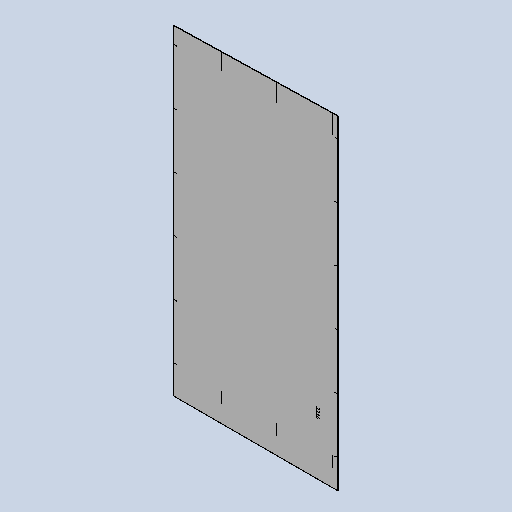
# Autodesk Inventor part: GBK 2231 shield 6
Saved by Autodesk Inventor 2026.2 (Build 302298010, 298A)
## iProperties
Created: 2026-04-17
Part Number: GBK 2231 shield 6
Material: Steel
Document SubType Name: Sheet Metal
Designer: pokla
Stock Number: 2236
Mass: 135011 g
Surface Area: 86345 cm^2
Volume: 17198.8 cm^3
Density: 7.85 g/cm^3
Flat Pattern Width: 148 cm
Flat Pattern Length: 292.2 cm
Flat Pattern Area: 43245.6 cm^2
Sheet Metal Rule: Default_mm
Sheet Metal Width: 1480,000 мм
Sheet Metal Length: 2922,000 мм
Sheet Metal Area: 4324560,000 мм^2
Appearance: Default
Author: admin
Autodesk Inventor part; units mm, degrees
ref_plane "YZ Plane" through (0, 0, 0) normal (1, 0, 0) x (0, 1, 0)
ref_plane "XZ Plane" through (0, 0, 0) normal (0, 1, 0) x (-1, 0, 0)
ref_plane "XY Plane" through (0, 0, 0) normal (0, 0, 1) x (1, 0, 0)
sketch "Sketch1" plane through (0, 0, 0) normal (0, 0, 1) x (1, 0, 0)
  line L0 (740, -1490) -> (-740, -1490)
  line L1 (-740, -1490) -> (-740, 1490)
  line L2 (-740, 1490) -> (740, 1490)
  line L3 (740, 1490) -> (740, -1490)
  line L4 (740, -1490) -> (-740, 1490) construction
  line L5 (-740, -1490) -> (740, 1490) construction
  line L6 (740, 1432) -> (-740, 1398.4141)
  point P0 (0, 0)
  dimension "d0" = 1480
  dimension "d1" = 2980
  dimension "d3" = 1.3
  dimension "d5" = 2922
  measures "d0" distance of L1.end L2.end
  measures "d1" distance of L0.end L1.end
  measures "d3" angle of L2 L6
  measures "d5" distance of L0.start L6.start
extrude "Plate1" add sketch "Sketch1" along normal blind 4 contours L0 L1 L6 L3
sketch "Sketch3" plane through (0, 0, 4) normal (0, 0, 1) x (1, 0, 0)
  line L0 (575.4966, -928.4274) -> (575.4966, -1128.991) construction
  line L1 (575.4966, -1128.991) -> (488.2456, -1128.991) construction
  line L2 (488.2456, -1128.991) -> (488.2456, -928.4274) construction
  line L3 (488.2456, -928.4274) -> (575.4966, -928.4274) construction
  line L4 (690.2486, -1238) -> (690.2486, -1335) projected
  line L5 (690.2486, -1335) -> (686.2496, -1335) projected
  line L6 (190.12, -1238) -> (190.12, -1335) projected
  line L7 (190.12, -1335) -> (186.121, -1335) projected
  line L8 (-310.0086, -1238) -> (-310.0086, -1335) projected
  line L9 (-310.0086, -1335) -> (-314.0076, -1335) projected
  line L10 (-310.0086, 1460.5) -> (-310.0086, 1256.8333) projected
  line L11 (190.12, 1460.5) -> (190.12, 1256.5) projected
  line L12 (690.2486, 1460.5) -> (690.2486, 1256.5) projected
  line L13 (770, 1252.8333) -> (710, 1252.8333) projected
  line L14 (710, 1248.8333) -> (710, 1252.8333) projected
  line L15 (770, 756.1667) -> (710, 756.1667) projected
  line L16 (710, 752.1667) -> (710, 756.1667) projected
  line L17 (770, 259.5) -> (710, 259.5) projected
  line L18 (710, 255.5) -> (710, 259.5) projected
  line L19 (770, -237.1667) -> (710, -237.1667) projected
  line L20 (710, -241.1667) -> (710, -237.1667) projected
  line L21 (770, -733.8333) -> (710, -733.8333) projected
  line L22 (710, -737.8333) -> (710, -733.8333) projected
  line L23 (770, -1230.5) -> (710, -1230.5) projected
  line L24 (710, -1234.5) -> (710, -1230.5) projected
  line L25 (-710, 1252.8333) -> (-739.3197, 1252.8333) projected
  line L26 (-710, 1248.8333) -> (-710, 1252.8333) projected
  line L27 (-710, 756.1667) -> (-739.3197, 756.1667) projected
  line L28 (-710, 752.1667) -> (-710, 756.1667) projected
  line L29 (-710, 259.5) -> (-739.3197, 259.5) projected
  line L30 (-710, 255.5) -> (-710, 259.5) projected
  line L31 (-710, -237.1667) -> (-739.3197, -237.1667) projected
  line L32 (-710, -241.1667) -> (-710, -237.1667) projected
  line L33 (-710, -733.8333) -> (-739.3197, -733.8333) projected
  line L34 (-710, -737.8333) -> (-710, -733.8333) projected
  line L35 (-710, -1230.5) -> (-739.3197, -1230.5) projected
  line L36 (-710, -1234.5) -> (-710, -1230.5) projected
  point P0 (0, 0)
  constraints: 2 other
mark "Mark2"
equation "\"d0\" = Лист_ширина"
equation "\"d2\" = Thickness"
equation "\"BendRadius\" = Thickness"
equation "\"BendReliefWidth\" = Thickness"
equation "\"BendReliefDepth\" = 0.5 * Thickness"
equation "\"CornerReliefSize\" = 4 * Thickness"
equation "\"MinimumRemnant\" = 2 * Thickness"
equation "\"TransitionRadius\" = BendRadius"
equation "\"JacobiRadiusSize\" = BendRadius"
equation "\"GapSize\" = Thickness"
equation "\"Лист_ширина\" = 1480"
equation "\"Thickness\" = 4"
body "Solid1"
